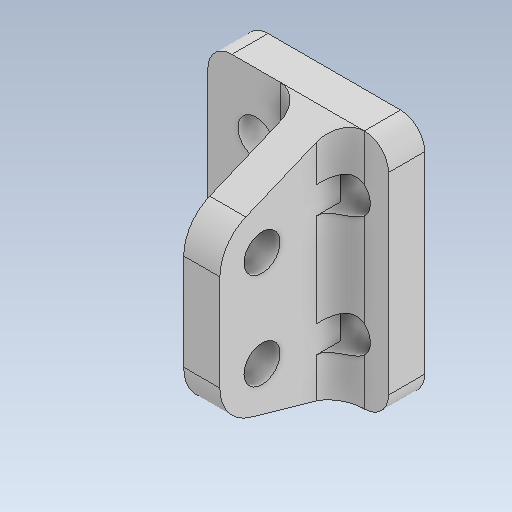
# Autodesk Inventor part: pcb_fixer_1
Saved by Autodesk Inventor 2020 (Build 240168000, 168)
## iProperties
Created: 2019-07-19
Part Number: pcb_fixer_1
Material: Generic
Document SubType Name: Modeling
Designer: psrob
Density: 1 g/cm^3
Appearance: Default
Author: psrob
Autodesk Inventor part; units mm, degrees
ref_plane "YZ Plane" through (0, 0, 0) normal (1, 0, 0) x (0, 1, 0)
ref_plane "XZ Plane" through (0, 0, 0) normal (0, 1, 0) x (-1, 0, 0)
ref_plane "XY Plane" through (0, 0, 0) normal (0, 0, 1) x (1, 0, 0)
sketch "Sketch1" plane through (0, 0, 0) normal (0, 0, 1) x (1, 0, 0)
  circle A0 centre (6, 16.5583) radius 1.5 projected
  circle A1 centre (7, -6.5583) radius 1.5 projected
  circle A2 centre (7, -26.5583) radius 1.5 projected
  circle A3 centre (15, -36.5583) radius 1.5 projected
  circle A4 centre (15, -16.5583) radius 1.5 projected
  circle A5 centre (14, 16.5583) radius 1.5 projected
  circle A6 centre (6, 26.5583) radius 1.5 projected
  circle A7 centre (14, 36.5583) radius 1.5 projected
  circle A8 centre (15, -6.5583) radius 1.5 projected
  circle A9 centre (15, -26.5583) radius 1.5 projected
  circle A10 centre (7, -36.5583) radius 1.5 projected
  circle A11 centre (7, -16.5583) radius 1.5 projected
  circle A12 centre (14, 26.5583) radius 1.5 projected
  circle A13 centre (6, 36.5583) radius 1.5 projected
  circle A14 centre (-6, 16.5583) radius 1.5 projected
  circle A15 centre (-7, -6.5583) radius 1.5 projected
  circle A16 centre (-7, -26.5583) radius 1.5 projected
  circle A17 centre (-15, -36.5583) radius 1.5 projected
  circle A18 centre (-15, -16.5583) radius 1.5 projected
  circle A19 centre (-14, 16.5583) radius 1.5 projected
  circle A20 centre (-6, 26.5583) radius 1.5 projected
  circle A21 centre (-14, 36.5583) radius 1.5 projected
  circle A22 centre (-15, -6.5583) radius 1.5 projected
  circle A23 centre (-15, -26.5583) radius 1.5 projected
  circle A24 centre (-7, -36.5583) radius 1.5 projected
  circle A25 centre (-7, -16.5583) radius 1.5 projected
  circle A26 centre (-14, 26.5583) radius 1.5 projected
  circle A27 centre (-6, 36.5583) radius 1.5 projected
  circle A28 centre (15.7386, 3.0583) radius 1.5 projected
  circle A29 centre (7.7386, 3.0583) radius 1.5 projected
  circle A30 centre (-15.7386, 3.0583) radius 1.5 projected
  circle A31 centre (-7.7386, 3.0583) radius 1.5 projected
  line L0 (17, 50.5583) -> (20, 47.5583) projected
  line L1 (-17, 50.5583) -> (17, 50.5583) projected
  line L2 (-20, 47.5583) -> (-17, 50.5583) projected
  line L3 (-20, -47.5583) -> (-20, 47.5583) projected
  line L4 (-17, -50.5583) -> (-20, -47.5583) projected
  line L5 (17, -50.5583) -> (-17, -50.5583) projected
  line L6 (20, -47.5583) -> (17, -50.5583) projected
  line L7 (20, 47.5583) -> (20, -47.5583) projected
  circle A32 centre (-7, 46.5583) radius 1.5 projected
  circle A33 centre (-14, 46.5583) radius 1.5 projected
  circle A34 centre (7, 46.5583) radius 1.5 projected
  circle A35 centre (14, 46.5583) radius 1.5 projected
  circle A36 centre (15, -46.5583) radius 1.5 projected
  circle A37 centre (7, -46.5583) radius 1.5 projected
  circle A38 centre (-15, -46.5583) radius 1.5 projected
  circle A39 centre (-7, -46.5583) radius 1.5 projected
  line L8 (-6, 16.5583) -> (-6, 11.5583)
  line L9 (-6, 11.5583) -> (-9, 11.5583)
  line L10 (-9, 11.5583) -> (-3, 11.5583)
  line L11 (-3, 11.5583) -> (-3, 31.5583)
  line L12 (-3, 31.5583) -> (-9, 31.5583)
  line L13 (-9, 31.5583) -> (-9, 11.5583)
  point P0 (0, 0)
  dimension "d0" = 5
  dimension "d1" = 3
  dimension "d2" = 6
  dimension "d3" = 20
  constraints: 12 end point, 2 parallel, 2 perpendicular, 1 horizontal, 1 vertical
  measures "d0" distance of L8.start L8.end
  measures "d1" distance of L8.end L9.end
  measures "d2" distance of L12.end L11.end
  measures "d3" distance of L11.end L10.end
extrude "Extrusion1" add sketch "Sketch1" along normal blind 3 contours L9 L13 L12 L11 L10
sketch "Sketch2" plane through (-9, 11.5583, 0) normal (-1, 0, 0) x (0, 0, 1)
  circle A0 centre (9.5, 13.5) radius 1.5 projected
  circle A1 centre (9.5, 5.5) radius 1.5 projected
  line L0 (3, 20) -> (3, 0) projected
  circle A2 centre (9.5, 5.5) radius 3.5
  circle A3 centre (9.5, 13.5) radius 3.5
  line L1 (9.5, 5.5) -> (13, 5.5)
  line L2 (13, 5.5) -> (13, 13.5)
  line L3 (9.5, 13.5) -> (13, 13.5)
  line L4 (3, 0) -> (10.4627, 2.135)
  line L5 (3, 20) -> (10.8462, 16.7308)
  line L6 (9.5, 13.5) -> (10.8462, 16.7308)
  line L7 (9.5, 5.5) -> (10.4627, 2.135)
  point P0 (0, -11.5583)
  dimension "d6" = 7
  dimension "d7" = 7
  constraints: 14 end point, 4 perpendicular, 4 point on circle, 2 centre point, 2 coincident, 2 tangent
  measures "d6" diameter of A2
  measures "d7" diameter of A3
ref_plane "Work Plane1" through (-10, -12.4417, 6) normal (1, 0, 0) x (0, 1, 0)
extrude "Extrusion2" add sketch "Sketch2" along normal up to surface (1 mm away) contours L3 A3 L6 A0 | A0 L6 A3 L3 | L2 A2 L4 L0 L5 A3 | L1 A1 L7 A2 | A2 L7 A1 L1
sketch "Sketch3" plane through (-9, 11.5583, 0) normal (-1, 0, 0) x (0, 0, 1)
  line L0 (22, -16.6525) -> (22, 10.6075) projected
  line L1 (8, 6.6225) -> (8, 7.7325) projected
  line L2 (0, 20) -> (0, 0) projected
  line L3 (0, 0) -> (3, 0) projected
  line L4 (3, 20) -> (3, 0) projected
  line L5 (0, 20) -> (3, 20) projected
  point P0 (0, -11.5583)
extrude "Extrusion3" add sketch "Sketch3" along normal up to surface (1 mm away)
sketch "Sketch4" plane through (-10, 11.5583, 0) normal (-1, 0, 0) x (0, 0, 1)
  line L0 (3, 0) -> (3, 20) projected
  line L1 (0, 20) -> (3, 20) projected
  line L2 (0, 0) -> (0, 20) projected
  line L3 (0, 0) -> (3, 0) projected
  point P0 (0, -11.5583)
extrude "Extrusion4" add sketch "Sketch4" along normal blind 8
sketch "Sketch5" plane through (-10, 11.5583, 3) normal (0, 0, 1) x (1, 0, 0)
  circle A0 centre (-4, 15) radius 1.5 projected
  circle A1 centre (-4, 5) radius 1.5 projected
  point P0 (10, -11.5583)
extrude "Extrusion5" cut sketch "Sketch5" against normal blind 8
thicken "Thicken1" operation add thickness 2 both sides no extend neighbours yes toward (1, 0, 0) faces at (-9, 22.6053, 4.6812)
fillet "Fillet1" radius 2 4 edges at (-7, 13.4993, 3) (-7, 21.5583, 3) (-7, 29.6173, 3) (-10, 21.5583, 3)
fillet "Fillet2" radius 2 4 edges at (-3, 31.5583, 1.5) (-3, 11.5583, 1.5) (-18, 31.5583, 1.5) (-18, 11.5583, 1.5)
body "Solid1"
